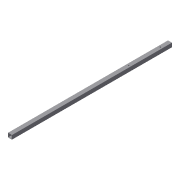
# Autodesk Inventor part: bpSupArm37
Saved by Autodesk Inventor 2017 (Build 210142000, 142)
## iProperties
Created: 2016-10-11
Part Number: bpSupArm37
Material: Generic
Document SubType Name: Modeling
Designer: krosie
Density: 1 g/cm^3
Appearance: Default
Author: krosie
Autodesk Inventor part; units mm, degrees
ref_plane "YZ Plane" through (0, 0, 0) normal (1, 0, 0) x (0, 1, 0)
ref_plane "XZ Plane" through (0, 0, 0) normal (0, 1, 0) x (-1, 0, 0)
ref_plane "XY Plane" through (0, 0, 0) normal (0, 0, 1) x (1, 0, 0)
sketch "Sketch2" plane through (0, 0, 0) normal (0, 0, 1) x (1, 0, 0)
  line L0 (-9.25, -9.5) -> (9.25, -9.5)
  line L1 (9.5, -9.25) -> (9.5, 9.25)
  line L2 (9.25, 9.5) -> (-9.25, 9.5)
  line L3 (-9.5, 9.25) -> (-9.5, -9.25)
  line L4 (-9.5, -9.5) -> (9.5, 9.5) construction
  line L5 (9.5, -9.5) -> (-9.5, 9.5) construction
  line L6 (-7.65, 7.9) -> (7.65, 7.9)
  line L7 (7.9, 7.65) -> (7.9, -7.65)
  line L8 (7.65, -7.9) -> (-7.65, -7.9)
  line L9 (-7.9, -7.65) -> (-7.9, 7.65)
  arc A0 (-9.25, 9.5) -> (-9.5, 9.25) centre (-9.25, 9.25) ccw
  arc A1 (-7.65, 7.9) -> (-7.9, 7.65) centre (-7.65, 7.65) ccw
  arc A2 (9.5, 9.25) -> (9.25, 9.5) centre (9.25, 9.25) ccw
  arc A3 (9.25, -9.5) -> (9.5, -9.25) centre (9.25, -9.25) ccw
  arc A4 (-9.5, -9.25) -> (-9.25, -9.5) centre (-9.25, -9.25) ccw
  arc A5 (-7.9, -7.65) -> (-7.65, -7.9) centre (-7.65, -7.65) ccw
  arc A6 (7.9, 7.65) -> (7.65, 7.9) centre (7.65, 7.65) ccw
  arc A7 (7.65, -7.9) -> (7.9, -7.65) centre (7.65, -7.65) ccw
  point P0 (0, 0)
  dimension "d0" = 19
  dimension "d1" = 19
  dimension "d2" = 1.6
  dimension "d3" = 0.25
  constraints: 20 end point, 16 point on circle, 16 tangent, 8 centre point, 8 point on line, 7 equal radius, 4 parallel, 2 midpoint, 2 perpendicular, 1 horizontal, 3 other
  measures "d0" distance of L5.end L4.end
  measures "d1" distance of L4.end L5.start
  measures "d2" distance between parallel lines of L2 L6
  measures "d3" radius of A0
extrude "Extrusion1" add sketch "Sketch2" against normal blind 760
sketch "Sketch3" plane through (-9.25, -9.5, 0) normal (0, -1, 0) x (1, 0, 0)
  circle A0 centre (9.25, -713.9463) radius 3.175 projected
  circle A1 centre (9.25, -563.9463) radius 3.175 projected
  point P0 (9.25, 0)
hole "Hole1" at (0, -9.5, -563.9463) at (0, -9.5, -713.9463) direction (0, 1, 0) diameter 5.5 end through all
sketch "Sketch5" plane through (-9.25, -9.5, 0) normal (0, -1, 0) x (1, 0, 0)
  circle A0 centre (9.25, -375.6475) radius 3 projected
  point P0 (9.25, 0)
hole "Hole2" at (0, -9.5, -375.6475) direction (0, 1, 0) diameter 6 end through all
body "Solid1"
